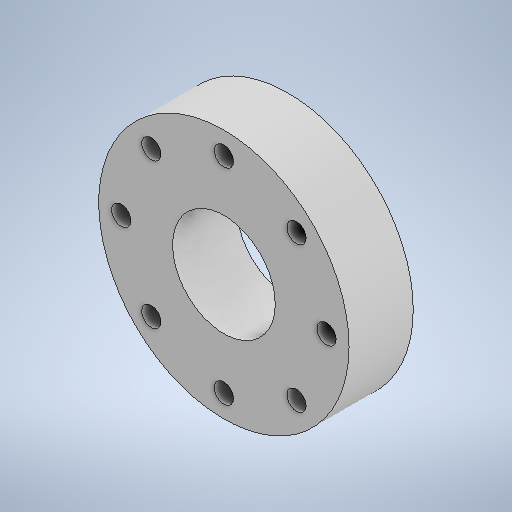
# Autodesk Inventor part: horn_3
Saved by Autodesk Inventor 2025.2 (Build 292293000, 293)
## iProperties
Created: 2025-02-13
Part Number: horn_3
Material: Generic
Document SubType Name: Modeling
Designer: Admin
Density: 1 g/cm^3
Appearance: Default
Author: Admin
Autodesk Inventor part; units mm, degrees
ref_plane "YZ Plane" through (0, 0, 0) normal (1, 0, 0) x (0, 1, 0)
ref_plane "XZ Plane" through (0, 0, 0) normal (0, 1, 0) x (-1, 0, 0)
ref_plane "XY Plane" through (0, 0, 0) normal (0, 0, 1) x (1, 0, 0)
sketch "Sketch2" plane through (0, 0, 0) normal (0, 0, 1) x (1, 0, 0)
  circle A0 centre (0, 8) radius 0.75
  circle A1 centre (0, 8) radius 0.75
  circle A2 centre (0, 0) radius 1
  circle A3 centre (-5.6569, 5.6569) radius 0.75
  circle A4 centre (-8, 0) radius 0.75
  circle A5 centre (-5.6569, -5.6569) radius 0.75
  circle A6 centre (0, -8) radius 0.75
  circle A7 centre (5.6569, -5.6569) radius 0.75
  circle A8 centre (8, 0) radius 0.75
  circle A9 centre (5.6569, 5.6569) radius 0.75
  circle A10 centre (0, 0) radius 9.75
  circle A11 centre (0, 0) radius 4
  point P0 (0.1028, -10.875)
  dimension "d5" = 360
  constraints: 12 centre point, 4 coincident, 17 other
extrude "Extrusion1" add sketch "Sketch2" along normal blind 5 contours A10
body "Solid1"
